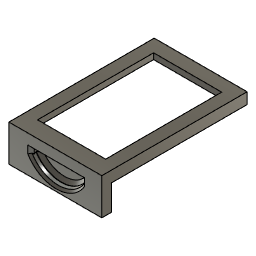
sdv1 (Autodesk Fusion 360 design; units mm, degrees)
Autodesk Fusion 360 part; units mm, degrees
sketch "Sketch1" plane through (0, 0, 0) normal (0, 0, 1) x (1, 0, 0)
  line L0 (0, 0) -> (24.5, 0)
  line L1 (24.5, 0) -> (24.5, 42)
  line L2 (24.5, 42) -> (0, 42)
  line L3 (0, 42) -> (0, 0)
  line L4 (5, 39.4) -> (20, 39.4)
  line L5 (20, 39.4) -> (20, 24.4)
  line L6 (20, 24.4) -> (5, 24.4)
  line L7 (5, 24.4) -> (5, 39.4)
  dimension "d1" = 24.5
  dimension "d2" = 42
  dimension "d3" = 15
  dimension "d4" = 15
  dimension "d5" = 5
  dimension "d6" = 2.6
  constraint horizontal L0
  constraint vertical L1
  constraint horizontal L2
  constraint vertical L3
  constraint coincident L0.start L3.end
  constraint horizontal L4
  constraint vertical L5
  constraint horizontal L6
  constraint vertical L7
  measures "d1" distance of L0.start L0.end
  measures "d2" distance of L0.start L2.end
  measures "d3" distance of L4.start L4.end
  measures "d4" distance of L4.start L6.end
  measures "d5" distance of L3 L7
  measures "d6" distance of L2 L4
extrude "Extrude1" add sketch "Sketch1" along normal blind 1.2 contours L0 L1 L2 L3 | L4 L5 L6 L7 makes body 1
extrude "Extrude2" add sketch "Sketch1" against normal blind 1.85 contours L4 L5 L6 L7 bodies 1
sketch "Sketch2" plane through (0, 42, 0) normal (0, 1, 0) x (-1, 0, 0)
  line L0 (-24.5, 0) -> (0, 0)
  line L1 (0, 0) -> (0, 1.2)
  line L2 (0, 1.2) -> (-24.5, 1.2)
  line L3 (-24.5, 1.2) -> (-24.5, 0)
  line L4 (-26.5, 3.2) -> (2, 3.2)
  line L5 (2, 3.2) -> (2, -8)
  line L6 (2, -8) -> (-26.5, -8)
  line L7 (-26.5, -8) -> (-26.5, 3.2)
  line L8 (-20, 0) -> (-5, 0)
  line L9 (-5, 0) -> (-5, -1.85)
  line L10 (-5, -1.85) -> (-20, -1.85)
  line L11 (-20, -1.85) -> (-20, 0)
  line L12 (-20.2, 0.2) -> (-4.8, 0.2)
  line L13 (-4.8, 0.2) -> (-4.8, -2.05)
  line L14 (-4.8, -2.05) -> (-20.2, -2.05)
  line L15 (-20.2, -2.05) -> (-20.2, 0.2)
  line L16 (-24.7, 1.4) -> (0.2, 1.4)
  line L17 (0.2, 1.4) -> (0.2, -0.2)
  line L18 (0.2, -0.2) -> (-24.7, -0.2)
  line L19 (-24.7, -0.2) -> (-24.7, 1.4)
  arc A0 (-20.2, -2.05) -> (-4.8, -2.05) centre (-12.5, 2.7935) ccw
  line L20 (-26.5, 1.4) -> (2, 1.4)
  line L21 (2, 1.4) -> (2, 3.2)
  line L22 (2, 3.2) -> (-26.5, 3.2)
  line L23 (-26.5, 3.2) -> (-26.5, 1.4)
  line L24 (0.2, -0.2) -> (2, -0.2)
  line L25 (2, -0.2) -> (2, 1.4)
  line L26 (2, 1.4) -> (0.2, 1.4)
  line L27 (0.2, 1.4) -> (0.2, -0.2)
  line L28 (-24.7, -0.2) -> (-26.5, -0.2)
  line L29 (-26.5, -0.2) -> (-26.5, 1.4)
  line L30 (-26.5, 1.4) -> (-24.7, 1.4)
  line L31 (-24.7, 1.4) -> (-24.7, -0.2)
  dimension "d11" = 2
  dimension "d12" = 8
  dimension "d13" = 2
  dimension "d14" = 2
  dimension "d15" = 0.2
  dimension "d16" = 0.2
  dimension "d17" = 0.2
  dimension "d18" = 0.2
  dimension "d19" = 0.2
  dimension "d20" = 0.2
  dimension "d21" = 0.2
  dimension "d22" = 0.2
  dimension "d27" = 9.0967
  dimension "d33" = 0.2
  constraint horizontal L4
  constraint vertical L5
  constraint horizontal L6
  constraint vertical L7
  constraint horizontal L8
  constraint vertical L9
  constraint horizontal L10
  constraint vertical L11
  constraint coincident L0 L8.start
  constraint horizontal L12
  constraint vertical L13
  constraint horizontal L14
  constraint vertical L15
  constraint horizontal L16
  constraint vertical L17
  constraint horizontal L18
  constraint vertical L19
  constraint horizontal L20
  constraint vertical L21
  constraint horizontal L22
  constraint vertical L23
  constraint coincident L7 L20.start
  constraint horizontal L24
  constraint vertical L25
  constraint horizontal L26
  constraint vertical L27
  constraint horizontal L28
  constraint vertical L29
  constraint horizontal L30
  constraint vertical L31
  measures "d11" distance of L2 L4
  measures "d12" distance of L0 L6
  measures "d13" distance of L3 L7
  measures "d14" distance of L1 L5
  measures "d15" distance of L9 L13
  measures "d16" distance of L11 L15
  measures "d17" distance of L8 L12
  measures "d18" distance of L10 L14
  measures "d19" distance of L3 L19
  measures "d20" distance of L2 L16
  measures "d21" distance of L1 L17
  measures "d22" distance of L0 L18
  measures "d27" radius of A0
  measures "d33" distance of L2 L20.start
extrude "Extrude3" add sketch "Sketch2" along normal blind 3 separate body contours L5 L6 L7 L13 L15 L18 A0 L24 L28 | L14 A0 | L7 L19 L20 L28 L29 L30 L31 | L5 L17 L20 L24 L25 L26 L27 | L4 L5 L7 L16 L20 L21 L22 L23 L26 L30 makes body 2
extrude "Extrude4" add sketch "Sketch2" along normal blind 0.4 contours L0 L8 L12 L13 L15 | L0 L1 L2 L3 L13 L15 L16 L17 L18 L19 L20 L27 L31 | L0 L1 L2 L3 L12 L13 L15 bodies 2
extrude "Extrude5" cut sketch "Sketch2" along normal blind 2.6 contours L14 A0 bodies 2
chamfer "Chamfer1" distance 1 angle 45 1 edges at (12.5, 44.6, -6.3032) on bodies 2
chamfer "Chamfer2" distance 1 angle 45 3 edges at (12.5, 42, -6.3032) (20.2, 42, -1.025) (4.8, 42, -1.025) on bodies 2
chamfer "Chamfer3" distance 0.5 angle 45 1 edges at (12.5, 43, -6.3032) on bodies 2
extrude "Extrude6" add sketch "Sketch2" along normal blind 44.6 contours L7 L19 L20 L28 L29 L30 L31 | L5 L17 L20 L24 L25 L26 L27 | L4 L5 L7 L16 L20 L21 L22 L23 L26 L30 bodies 2
sketch "Sketch3" plane through (0, 0, 1.4) normal (0, 0, -1) x (1, 0, 0)
  line L0 (24.7, -42.4) -> (-0.2, -42.4)
  line L1 (-0.2, -42.4) -> (-0.2, -86.6)
  line L2 (-0.2, -86.6) -> (24.7, -86.6)
  line L3 (24.7, -86.6) -> (24.7, -42.4)
  line L4 (-0.2, -86.6) -> (24.7, -86.6)
  line L5 (24.7, -86.6) -> (24.7, -84.6)
  line L6 (24.7, -84.6) -> (-0.2, -84.6)
  line L7 (-0.2, -84.6) -> (-0.2, -86.6)
  line L8 (1.8, -47) -> (22.7, -47)
  line L9 (22.7, -47) -> (22.7, -82.6)
  line L10 (22.7, -82.6) -> (1.8, -82.6)
  line L11 (1.8, -82.6) -> (1.8, -47)
  line L12 (26.5, -45) -> (-2, -45)
  dimension "d36" = 2
  dimension "d37" = 2
  dimension "d38" = 2
  dimension "d39" = 2
  dimension "d40" = 2
  constraint horizontal L4
  constraint vertical L5
  constraint horizontal L6
  constraint vertical L7
  constraint coincident L1.end L2.start
  constraint horizontal L8
  constraint vertical L9
  constraint horizontal L10
  constraint vertical L11
  measures "d36" distance of L1.end L6.end
  measures "d37" distance of L8 L12
  measures "d38" distance of L3 L9
  measures "d39" distance of L1 L11
  measures "d40" distance of L6 L10
extrude "Extrude7" add sketch "Sketch3" along normal blind 1.6 contours L1 L2 L3 L4 L5 L6 L7 bodies 2
extrude "Extrude8" cut sketch "Sketch3" against normal blind 10 contours L8 L9 L10 L11 bodies 2
hidden bodies 1
equation "d34 = 42 mm + 0.6 mm + 2 mm"
